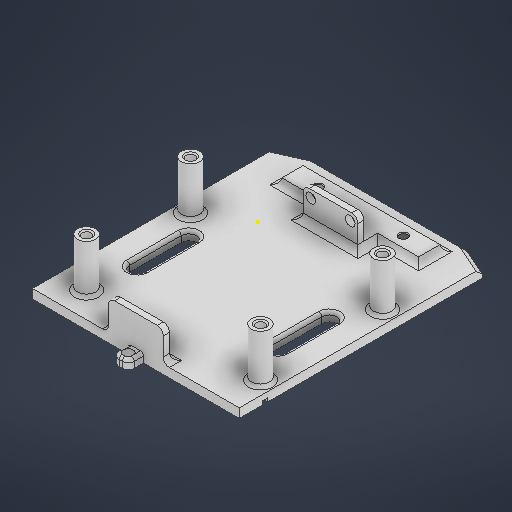
# Autodesk Inventor part: PodstawaTrojkolowa
Saved by Autodesk Inventor 2026 (Build 300175000, 175)
## iProperties
Created: 2025-04-23
Part Number: PodstawaTrojkolowa
Material: Generic
Document SubType Name: Modeling
Designer: isan
Density: 1 g/cm^3
Appearance: Default
Author: isan
Autodesk Inventor part; units mm, degrees
ref_plane "YZ Plane" through (0, 0, 0) normal (1, 0, 0) x (0, 1, 0)
ref_plane "XZ Plane" through (0, 0, 0) normal (0, 1, 0) x (-1, 0, 0)
ref_plane "XY Plane" through (0, 0, 0) normal (0, 0, 1) x (1, 0, 0)
sketch "Sketch2" plane through (0, 0, 0) normal (0, 1, 0) x (-1, 0, 0)
  line L0 (-34, 40) -> (34, 40)
  line L1 (34, 40) -> (34, -40)
  line L2 (34, -40) -> (-34, -40)
  line L3 (-34, -40) -> (-34, 40)
  line L4 (-34, 40) -> (34, -40) construction
  line L5 (34, 40) -> (-34, -40) construction
  point P0 (0, 0)
  dimension "d5" = 80
  dimension "d6" = 68
  constraints: 12 end point, 2 midpoint, 2 parallel, 1 horizontal, 1 perpendicular
  measures "d5" distance of L0.end L1.end
  measures "d6" distance of L1.end L2.end
extrude "Extrusion1" add sketch "Sketch2" along normal blind 3
sketch "Sketch3" plane through (0, 3, 0) normal (0, 1, 0) x (1, 0, 0)
  line L0 (-23.1, 0.5) -> (-23.1, -16.5) construction
  line L1 (-25.6, 0.5) -> (-25.6, -16.5)
  line L2 (-20.6, -16.5) -> (-20.6, 0.5)
  arc A0 (-20.6, 0.5) -> (-25.6, 0.5) centre (-23.1, 0.5) ccw
  arc A1 (-25.6, -16.5) -> (-20.6, -16.5) centre (-23.1, -16.5) ccw
  line L3 (-34, 40) -> (-34, -40) projected
  line L4 (-40.9526, -8) -> (2.3583, -8)
  point P0 (0, 0)
  point P1 (-23.1, -8)
  point P2 (-23.1, 3)
  point P3 (-23.1, -19)
  point P4 (-25.6, -8)
  dimension "d9" = 22
  dimension "d12" = 2.5
  dimension "d13" = 8.4
  dimension "d181" = 8
  constraints: 10 end point, 6 point on circle, 4 tangent, 2 centre point, 2 midpoint, 1 horizontal, 1 parallel, 1 point on line, 1 vertical
  measures "d9" distance of point (-23.1, 3) point (-23.1, -19)
  measures "d12" radius of A0
  measures "d13" distance from line of L3 point (-25.6, -8)
  measures "d181" distance from line of L4 point (0, 0)
extrude "Extrusion2" cut sketch "Sketch3" against normal blind 3
mirror "Mirror1" about plane through (0, 0, 0) normal (1, 0, 0) of "Extrusion2"
sketch "Sketch4" plane through (0, 3, 0) normal (0, 1, 0) x (1, 0, 0)
  circle A0 centre (-29.6, 7.557) radius 3
  line L0 (-34, 40) -> (-34, -40) projected
  line L1 (-34, -40) -> (34, -40) projected
  line L2 (34, 40) -> (-34, 40) projected
  circle A1 centre (29.583, -28.6) radius 3
  line L3 (34, -40) -> (34, 40) projected
  circle A2 centre (29.525, 11.595) radius 3
  circle A3 centre (-24.6, -31.6) radius 3
  point P0 (0, 0)
  dimension "d23" = 6
  dimension "d28" = 6
  dimension "d31" = 6
  dimension "d34" = 6
  dimension "d65" = 29.6
  dimension "d66" = 7.557
  dimension "d67" = 29.525
  dimension "d68" = 11.595
  dimension "d69" = 28.6
  dimension "d70" = 29.583
  dimension "d71" = 31.6
  dimension "d72" = 24.6
  constraints: 4 centre point
  measures "d23" diameter of A0
  measures "d28" diameter of A1
  measures "d31" diameter of A2
  measures "d34" diameter of A3
  measures "d65" horizontal distance of point (0, 0) A0.centre
  measures "d66" vertical distance of point (0, 0) A0.centre
  measures "d67" horizontal distance of point (0, 0) A2.centre
  measures "d68" vertical distance of point (0, 0) A2.centre
  measures "d69" vertical distance of point (0, 0) A1.centre
  measures "d70" horizontal distance of point (0, 0) A1.centre
  measures "d71" vertical distance of A3.centre point (0, 0)
  measures "d72" horizontal distance of point (0, 0) A3.centre
extrude "Extrusion3" add sketch "Sketch4" along normal blind 16 contours A0 | A1 | A2 | A3
sketch "Sketch5" plane through (0, 3, 0) normal (0, 1, 0) x (1, 0, 0)
  line L0 (9, 26) -> (-9, 26)
  line L1 (-9, 26) -> (-9, 24)
  line L2 (-9, 24) -> (9, 24)
  line L3 (9, 24) -> (9, 26)
  line L4 (9, -38) -> (-9, -38)
  line L5 (-9, -38) -> (-9, -40)
  line L6 (-9, -40) -> (9, -40)
  line L7 (9, -40) -> (9, -38)
  line L8 (-34, -40) -> (34, -40) projected
  point P0 (0, 0)
  point P1 (0, 24)
  point P2 (9, -39)
  point P3 (-9, -39)
  point P4 (0, -38)
  dimension "d163" = 18
  dimension "d164" = 9
  dimension "d166" = 2
  dimension "d167" = 2
  dimension "d168" = 18
  dimension "d169" = 9
  dimension "d171" = 62
  constraints: 16 end point, 4 midpoint, 4 parallel, 2 horizontal, 2 perpendicular, 1 collinear
  measures "d163" distance of L0.start L0.end
  measures "d164" distance from line of point (0, 0) L3
  measures "d166" distance of L2.end L0.start
  measures "d167" distance of L6.end L4.start
  measures "d168" distance of L5.end L6.end
  measures "d169" horizontal distance of point (0, 0) point (9, -39)
  measures "d171" distance of point (0, -38) point (0, 24)
extrude "Extrusion4" add sketch "Sketch5" along normal blind 10
sketch "Sketch6" plane through (-29.6, 19, -7.557) normal (0, 1, 0) x (1, 0, 0)
  point P0 (29.6, -7.557)
sketch "Sketch7" plane through (-29.6, 19, -7.557) normal (0, 1, 0) x (1, 0, 0)
  circle A0 centre (0, 0) radius 1.5
  circle A1 centre (0, 0) radius 3 projected
  point P0 (29.6, -7.557)
  dimension "d44" = 3
  constraints: 1 centre point, 1 coincident
  measures "d44" diameter of A0
extrude "Extrusion5" cut sketch "Sketch7" against normal blind 10 contours A0
sketch "Sketch8" plane through (29.525, 19, -11.595) normal (0, 1, 0) x (1, 0, 0)
  circle A0 centre (0, 0) radius 1.5
  point P0 (-29.525, -11.595)
  dimension "d48" = 3
  constraints: 1 centre point
  measures "d48" diameter of A0
extrude "Extrusion6" cut sketch "Sketch8" against normal blind 10
sketch "Sketch9" plane through (-24.6, 19, 31.6) normal (0, 1, 0) x (1, 0, 0)
  circle A0 centre (0, 0) radius 3 projected
  circle A1 centre (0, 0) radius 1.5
  circle A2 centre (54.183, 3) radius 1.5
  circle A3 centre (54.183, 3) radius 3 projected
  point P0 (24.6, 31.6)
  dimension "d51" = 3
  dimension "d52" = 3
  constraints: 2 centre point, 2 coincident
  measures "d51" diameter of A1
  measures "d52" diameter of A2
extrude "Extrusion7" cut sketch "Sketch9" against normal blind 10 contours A1 | A2
sketch "Sketch11" plane through (0, 0, 0) normal (0, -1, 0) x (1, 0, 0)
  line L0 (-34, 32.4) -> (-12.3, 32.4)
  line L1 (-12.3, 32.4) -> (-12.3, 30.6)
  line L2 (-12.3, 30.6) -> (-34, 30.6)
  line L3 (-34, 30.6) -> (-34, 32.4)
  line L4 (-34, -40) -> (-34, 40) projected
  line L5 (-34, 40) -> (34, 40) projected
  point P0 (0, 0)
  point P1 (-34, 31.5)
  dimension "d60" = 1.8
  dimension "d61" = 21.7
  dimension "d62" = 8.5
  constraints: 8 end point, 2 parallel, 1 collinear, 1 horizontal, 1 midpoint, 1 perpendicular
  measures "d60" distance of L0.end L1.end
  measures "d61" distance of L1.end L2.end
  measures "d62" distance from line of L5 point (-34, 31.5)
extrude "Extrusion9" cut sketch "Sketch11" against normal blind 1.2
mirror "Mirror6" about plane through (0, 0, 0) normal (1, 0, 0) of "Extrusion9"
chamfer "Chamfer3" distance 0.4 angle 45 4 edges at (-31.1, 19, -7.557) (28.025, 19, -11.595) (28.083, 19, 28.6) (-26.1, 19, 31.6)
sketch "Sketch12" plane through (0, 0, 0) normal (0, -1, 0) x (1, 0, 0)
  line L0 (0, -50.2706) -> (0, 0) construction
  line L1 (34, -40) -> (-34, -40) projected
  line L2 (-2.5, 45) -> (2.5, 45)
  line L3 (2.5, 45) -> (2.5, 40)
  line L4 (2.5, 40) -> (-2.5, 40)
  line L5 (-2.5, 40) -> (-2.5, 45)
  line L6 (-2.5, 45) -> (2.5, 40) construction
  line L7 (2.5, 45) -> (-2.5, 40) construction
  circle A0 centre (0, 42.5) radius 1.575
  line L8 (7, 40) -> (-7, 40) projected
  line L9 (0, 41.2812) -> (0, 0) construction
  point P0 (2.5, -33)
  dimension "d82" = 5
  dimension "d83" = 5
  dimension "d84" = 3.15
  constraints: 16 end point, 2 collinear, 2 midpoint, 2 parallel, 1 centre point, 1 coincident, 1 perpendicular, 1 point on line, 1 vertical
  measures "d82" distance of L2.end L3.end
  measures "d83" distance of L2.start L2.end
  measures "d84" diameter of A0
extrude "Extrusion10" add sketch "Sketch12" against normal blind 3
fillet "Fillet2" radius 2 2 edges at (2.5, 1.5, 45) (-2.5, 1.5, 45)
fillet "Fillet3" radius 1 5 edges at (0, 3, 45) (-1.9142, 3, 44.4142) (-2.5, 3, 41.5) (2.5, 3, 41.5) (1.9142, 3, 44.4142)
sketch "Sketch13" plane through (0, 0, 0) normal (0, -1, 0) x (1, 0, 0)
  line L0 (-34, 40) -> (34, 40) projected
  line L1 (25, -44) -> (-25, -44)
  line L2 (-25, -44) -> (-25, -40)
  line L3 (-25, -40) -> (25, -40)
  line L4 (25, -40) -> (25, -44)
  line L5 (25, -44) -> (-25, -40) construction
  line L6 (-25, -44) -> (25, -40) construction
  line L7 (25, -44) -> (34, -40)
  line L8 (-25, -44) -> (-34, -40)
  line L9 (7, -40) -> (-7, -40) projected
  line L10 (0, 0) -> (0, -49.5761) construction
  line L11 (34, -40) -> (-34, -40)
  point P0 (0, -42)
  point P1 (-34, -40)
  dimension "d92" = 4
  dimension "d93" = 50
  constraints: 20 end point, 2 coincident, 2 midpoint, 2 parallel, 1 collinear, 1 horizontal, 1 perpendicular, 1 point on line, 1 vertical
  measures "d92" distance of L3.end L1.start
  measures "d93" distance of L1.start L1.end
fillet "Face Fillet5" radius 1 1 edges at (26.583, 3, 28.6)
fillet "Face Fillet6" radius 1 1 edges at (26.525, 3, -11.595)
fillet "Face Fillet7" radius 1 1 edges at (-32.6, 3, -7.557)
fillet "Face Fillet8" radius 1 1 edges at (-27.6, 3, 31.6)
fillet "Fillet4" radius 1 8 edges at (-23.1, 3, 19) (-25.6, 3, 8) (-23.1, 3, -3) (-20.6, 3, 8) (23.1, 3, -3) (25.6, 3, 8) (23.1, 3, 19) (20.6, 3, 8)
extrude "Extrusion14" add sketch "Sketch13" against normal blind 3
chamfer "Chamfer5" distance 2 angle 45 3 edges at (0, 3, -44) (29.5, 3, -42) (-29.5, 3, -42)
sketch "Sketch18" plane through (0, 0, 0) normal (0, -1, 0) x (1, 0, 0)
  circle A0 centre (0, -28) radius 6.2
  line L0 (0, -24.0708) -> (0, 69.4783) construction
  line L1 (0.9, -20.5) -> (-0.9, -20.5)
  line L2 (-0.9, -20.5) -> (-0.9, -35.5)
  line L3 (-0.9, -35.5) -> (0.9, -35.5)
  line L4 (0.9, -35.5) -> (0.9, -20.5)
  line L5 (0.9, -20.5) -> (-0.9, -35.5) construction
  line L6 (-0.9, -20.5) -> (0.9, -35.5) construction
  point P0 (0, 0)
  point P1 (0.9, -34.1343)
  point P2 (0.9, -21.8657)
  point P3 (-0.9, -21.8657)
  point P4 (-0.9, -34.1343)
  dimension "d157" = 12.4
  dimension "d158" = 28
  dimension "d159" = 1.8
  dimension "d160" = 15
  constraints: 14 end point, 2 midpoint, 2 parallel, 2 point on line, 1 centre point, 1 horizontal, 1 perpendicular, 1 vertical
  measures "d157" diameter of A0
  measures "d158" distance of point (0, 0) A0.centre
  measures "d159" distance of L2.end L3.end
  measures "d160" distance of L1.end L2.end
extrude "Extrusion17" cut sketch "Sketch18" against normal blind 1.1 contours L4 A0 L2
sketch "Sketch20" plane through (0, 3, 0) normal (0, 1, 0) x (1, 0, 0)
  circle A0 centre (-14, 34) radius 1.5
  line L0 (-34, 37.8114) -> (-34, -40) projected
  line L1 (25, 44) -> (-25, 44) projected
  point P0 (0, 0)
  dimension "d182" = 3
  dimension "d183" = 20
  dimension "d184" = 10
  constraints: 1 centre point
  measures "d182" diameter of A0
  measures "d183" distance from line of L0 A0.centre
  measures "d184" distance from line of L1 A0.centre
extrude "Extrusion19" cut sketch "Sketch20" against normal blind 3
sketch "Sketch23" plane through (0, 3, 0) normal (0, 1, 0) x (1, 0, 0)
  circle A0 centre (-14, 34) radius 1.5 projected
  circle A1 centre (-14, 34) radius 2.75
  point P0 (0, 0)
  dimension "d193" = 5.5
  constraints: 1 centre point, 1 coincident
  measures "d193" diameter of A1
extrude "Extrusion22" cut sketch "Sketch23" against normal blind 2.6 contours A0 | A1
sketch "Sketch24" plane through (0, 3, 0) normal (0, 1, 0) x (1, 0, 0)
  line L0 (-22.5, 30.5) -> (22.5, 30.5)
  line L1 (22.5, 30.5) -> (22.5, 37.5)
  line L2 (22.5, 37.5) -> (-22.5, 37.5)
  line L3 (-22.5, 37.5) -> (-22.5, 30.5)
  line L4 (-24.5756, 42) -> (24.5756, 42) projected
  circle A0 centre (-14, 34) radius 2.75 projected
  line L5 (-14, 34) -> (-5.2691, 34)
  point P0 (0, 0)
  point P1 (0, 42)
  point P2 (-22.5, 34)
  dimension "d196" = 45
  dimension "d197" = 7
  dimension "d198" = 22.5
  constraints: 10 end point, 2 horizontal, 2 midpoint, 2 parallel, 1 perpendicular, 1 point on line
  measures "d196" distance of L0.start L0.end
  measures "d197" distance of L2.end L0.start
  measures "d198" distance from line of point (0, 42) L3
extrude "Extrusion23" add sketch "Sketch24" along normal blind 2
sketch "Sketch26" plane through (0, 5, 0) normal (0, 1, 0) x (1, 0, 0)
  circle A0 centre (-14, 34) radius 2.75 projected
  circle A1 centre (-14, 34) radius 1.5
  circle A2 centre (-14, 34) radius 2.75
  point P0 (0, 0)
  constraints: 2 centre point, 2 coincident, 1 concentric
extrude "Extrusion24" add sketch "Sketch26" against normal blind 0.4
mirror "Mirror14" about plane through (0, 0, 0) normal (1, 0, 0) of "Extrusion19"
mirror "Mirror15" about plane through (0, 0, 0) normal (1, 0, 0) of "Extrusion22"
sketch "Sketch27" plane through (0, 5, 0) normal (0, 1, 0) x (1, 0, 0)
  circle A0 centre (14, 34) radius 1.5 projected
  circle A1 centre (14, 34) radius 1.5
  point P0 (0, 0)
  constraints: 1 centre point, 1 coincident
extrude "Extrusion25" cut sketch "Sketch27" against normal blind 2
sketch "Sketch28" plane through (14, 3, -34) normal (0, -1, 0) x (1, 0, 0)
  circle A0 centre (0, 0) radius 1.5 projected
  circle A1 centre (0, 0) radius 2.75
  point P0 (-14, 34)
  dimension "d205" = 5.5
  constraints: 1 centre point, 1 coincident
  measures "d205" diameter of A1
extrude "Extrusion26" cut sketch "Sketch28" against normal blind 1.6 contours A0 | A1
sketch "Sketch29" plane through (0, 3, 0) normal (0, 1, 0) x (1, 0, 0)
  line L0 (9, 26) -> (11, 28) projected
  line L1 (9, 26) -> (-9, 26)
  line L2 (-9, 26) -> (-9, 30.5)
  line L3 (-9, 30.5) -> (9, 30.5)
  line L4 (9, 30.5) -> (9, 26)
  line L5 (-22.5, 30.5) -> (22.5, 30.5) projected
  line L6 (-9, 26) -> (-9, 24) projected
  line L7 (9, 24) -> (9, 26) projected
  point P0 (0, 0)
  constraints: 8 end point, 3 collinear, 2 parallel, 1 horizontal, 1 perpendicular
extrude "Extrusion27" add sketch "Sketch29" along normal blind 2
sketch "Sketch30" plane through (9, 13, -26) normal (0, 0, -1) x (-1, 0, 0)
  circle A0 centre (2.5, -2.5) radius 1.6
  line L0 (0, 0) -> (18, 0) projected
  line L1 (0, -8) -> (0, 0) projected
  point P0 (9, -13)
  dimension "d210" = 3.2
  dimension "d211" = 2.5
  dimension "d212" = 2.5
  constraints: 1 centre point
  measures "d210" diameter of A0
  measures "d211" distance from line of L0 A0.centre
  measures "d212" distance from line of L1 A0.centre
extrude "Extrusion28" cut sketch "Sketch30" against normal blind 2
mirror "Mirror17" about plane through (0, 0, 0) normal (1, 0, 0) of "Extrusion28"
fillet "Fillet7" radius 2 2 edges at (-9, 13, -25) (9, 13, -25)
fillet "Fillet8" radius 2 5 edges at (0, 3, 38) (-9, 3, 39) (9, 3, 39) (-9, 13, 39) (9, 13, 39)
fillet "Fillet9" radius 2 8 edges at (0, 3, -37.5) (-15.75, 3, -30.5) (-22.5, 3, -34) (22.5, 3, -34) (9, 3, -27.25) (15.75, 3, -30.5) (0, 3, -24) (-9, 3, -27.25)
body "Solid1"
